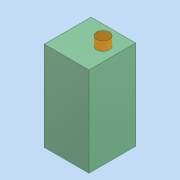
# Autodesk Inventor part: arduino_radio_volume
Saved by Autodesk Inventor 2020.3 (Build 243373000, 373)
## iProperties
Created: 2020-06-02
Part Number: arduino_radio_volume
Material: ABS Plastic
Document SubType Name: Modeling
Designer: Derek Wider
Density: 1.06 g/cm^3
Appearance: Smooth - Dark Sea Green
Author: Derek Wider
Autodesk Inventor part; units mm, degrees
ref_plane "YZ Plane" through (0, 0, 0) normal (1, 0, 0) x (0, 1, 0)
ref_plane "XZ Plane" through (0, 0, 0) normal (0, 1, 0) x (-1, 0, 0)
ref_plane "XY Plane" through (0, 0, 0) normal (0, 0, 1) x (1, 0, 0)
sketch "Sketch1" plane through (0, 0, 0) normal (0, 1, 0) x (-1, 0, 0)
  line L0 (0, 0) -> (22.098, 0)
  line L1 (22.098, 0) -> (22.098, -23.114)
  line L2 (22.098, -23.114) -> (0, -23.114)
  line L3 (0, -23.114) -> (0, 0)
  dimension "d0" = 22.098
  dimension "d1" = 23.114
  constraints: 8 end point, 2 parallel, 1 horizontal, 1 perpendicular
  measures "d0" distance of L1.end L2.end
  measures "d1" distance of L0.end L1.end
extrude "Extrusion1" add sketch "Sketch1" along normal blind 44.196
sketch "Sketch2" plane through (0, 44.196, 0) normal (0, 1, 0) x (1, 0, 0)
  circle A0 centre (-6.7327, 13.6931) radius 3.175
  point P0 (0, 0)
  dimension "d4" = 6.35
  constraints: 1 centre point
  measures "d4" diameter of A0
extrude "Extrusion2" add sketch "Sketch2" along normal blind 4.445
body "Solid1"
